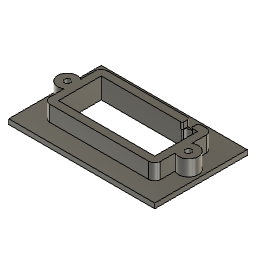
Servo support aileron v3 (Autodesk Fusion 360 design; units mm, degrees)
Autodesk Fusion 360 part; units mm, degrees
note: some values were not read from the file. Chosen so that the rebuilt part matches the saved one: which face or edge a step refers to. Set by a fixed rule: which sketch regions a step uses.
sketch "Sketch1" plane through (0, 0, 0) normal (0, 0, 1) x (1, 0, 0)
  line L0 (11.6, 5.15) -> (-11.6, 5.15)
  line L1 (-11.6, 5.15) -> (-11.6, -5.15)
  line L2 (-11.6, -5.15) -> (11.6, -5.15)
  line L3 (11.6, -5.15) -> (11.6, 5.15)
  line L4 (11.6, 5.15) -> (-11.6, -5.15) construction
  line L5 (-11.6, 5.15) -> (11.6, -5.15) construction
  line L6 (-17.6, -11.15) -> (17.6, -11.15)
  line L7 (17.6, -11.15) -> (17.6, 11.15)
  line L8 (17.6, 11.15) -> (-17.6, 11.15)
  line L9 (-17.6, 11.15) -> (-17.6, -11.15)
  line L10 (13.4, 6.95) -> (-13.4, 6.95)
  line L11 (-13.4, 6.95) -> (-13.4, -6.95)
  line L12 (-13.4, -6.95) -> (13.4, -6.95)
  line L13 (13.4, -6.95) -> (13.4, 6.95)
  dimension "d1" = 23.2
  dimension "d2" = 10.3
  dimension "d3" = 6
  dimension "d4" = 1.8
  constraint horizontal L0
  constraint perpendicular L0 L1
  constraint parallel L0 L2
  constraint parallel L1 L3
  constraint coincident L4 origin
  constraint coincident L5 origin
  measures "d1" distance of L1.end L2.end
  measures "d2" distance of L0.end L1.end
extrude "Extrude1" add sketch "Sketch1" along normal blind 7 contours L10 L11 L12 L13
extrude "Extrude2" add sketch "Sketch1" along normal blind 1.2 contours L6 L7 L8 L9
sketch "Sketch2" plane through (0, 0, 0) normal (0, 0, 1) x (1, 0, 0)
  line L0 (-22, 0) -> (23, 0) construction
  circle A0 centre (14.6, 0) radius 0.75 construction
  line L1 (11.6, -5.15) -> (11.6, 5.15) construction
  dimension "d9" = 1.5
  dimension "d10" = 3
  constraint horizontal L0
  constraint coincident L0 A0.centre
  measures "d9" diameter of A0
  measures "d10" distance of A0.centre L1
sketch "Sketch3" plane through (0, 0, 1.2) normal (0, 0, 1) x (-1, 0, 0)
  line L0 (-13.4, -6.95) -> (-13.4, 6.95)
  line L1 (-13.4, 6.95) -> (13.4, 6.95)
  line L2 (13.4, 6.95) -> (13.4, -6.95)
  line L3 (13.4, -6.95) -> (-13.4, -6.95)
  line L4 (17.6, -11.15) -> (17.6, 11.15)
  line L5 (17.6, 11.15) -> (-17.6, 11.15)
  line L6 (-17.6, 11.15) -> (-17.6, -11.15)
  line L7 (-17.6, -11.15) -> (17.6, -11.15)
  circle A0 centre (-14.6, 0) radius 0.75
  circle A1 centre (-14.6, 0) radius 2.35
  dimension "d11" = 1.6
extrude "Extrude3" add sketch "Sketch3" along normal blind 5 contours L0 A1 picked at (-13.55, 0)
extrude "Extrude9" cut 1 faces at (14.8389, -0.0008, 1.2) along direction (0, 0, -1) up to surface (1.2 mm away)
mirror "Mirror1" about plane through (0, 0, 0) normal (1, 0, 0) of "Extrude2", "Extrude3"
sketch "Sketch4" plane through (0, 0, 0) normal (0, 0, 1) x (1, 0, 0)
  line L0 (11.6, -1) -> (17.6, -1)
  line L1 (17.6, -1) -> (17.6, 0.9)
  line L2 (17.6, 0.9) -> (11.6, 0.9)
  line L3 (11.6, 0.9) -> (11.6, -1)
  constraint horizontal L0
  constraint vertical L1
  constraint horizontal L2
  constraint vertical L3
sketch "Sketch5" plane through (0, 0, 0) normal (0, 0, 1) x (1, 0, 0)
  arc A0 (10.0479, 5.1477) -> (7.9479, 5.146) centre (8.9979, 5.148) ccw
  line L0 (7.9479, 5.146) -> (10.0479, 5.1477)
  dimension "d17" = 1.05
  measures "d17" radius of A0
extrude "Extrude4" cut sketch "Sketch5" along normal up to surface (7 mm away)
extrude "Extrude5" add 2 faces at (13.55, 0, 6.2) (-13.55, 0, 6.2) along direction (0, 0, 1) up to surface end surface through (0, 0, 7) normal (0, 0, 1) offset 0
sketch "Sketch6" plane through (0, 0, 7) normal (0, 0, 1) x (-1, 0, 0)
  circle A0 centre (14.6, 0) radius 0.75
  circle A1 centre (-14.6, 0) radius 0.75
  line L0 (-13.4, 6.95) -> (-13.4, 2.0205)
  arc A2 (-13.4, 2.0205) -> (-13.4, -2.0205) centre (-14.6, 0) ccw
  line L1 (-13.4, -2.0205) -> (-13.4, -6.95)
  line L2 (-13.4, -6.95) -> (13.4, -6.95)
  line L3 (13.4, -6.95) -> (13.4, -2.0205)
  arc A3 (13.4, -2.0205) -> (13.4, 2.0205) centre (14.6, 0) ccw
  line L4 (13.4, 2.0205) -> (13.4, 6.95)
  line L5 (13.4, 6.95) -> (-13.4, 6.95)
  arc A4 (-10.0479, -5.15) -> (-7.9479, -5.15) centre (-8.9979, -5.148) ccw
  line L6 (-10.0479, -5.15) -> (-11.6, -5.15)
  line L7 (-11.6, -5.15) -> (-11.6, 5.15)
  line L8 (-11.6, 5.15) -> (11.6, 5.15)
  line L9 (11.6, 5.15) -> (11.6, -5.15)
  line L10 (11.6, -5.15) -> (-7.9479, -5.15)
  line L11 (-10.0479, -5.15) -> (-10.0444, -6.95)
  line L12 (-7.9479, -5.15) -> (-7.9514, -6.95)
  constraint coincident A4.start L6.start
  constraint coincident L2 L11.end
  constraint tangent A4 L11
  constraint coincident A4.end L10.end
  constraint coincident L2 L12.end
  constraint tangent A4 L12
extrude "Extrude6" cut sketch "Sketch6" against normal blind 1.5 contours L2 A4 L11 L12
extrude "Extrude7" cut 1 faces at (8.9718, 6.6983, 5.5) along direction (0, 0, -1) blind 2
extrude "Extrude8" cut 1 faces at (-3.8667, -6.35, 7) along direction (0, 0, -1) blind 2
fillet "Fillet1" radius 0.35 2 edges at (7.9479, 5.15, 2.75) (10.0479, 5.15, 2.75)
fillet "Fillet2" radius 1.5 4 edges at (-13.4, 6.95, 3.1) (13.4, 6.95, 3.1) (-13.4, -6.95, 3.1) (13.4, -6.95, 3.1)
fillet "Fillet5" radius 0.5 3 edges at (8.9979, 6.95, 3.5) (7.9514, 6.95, 4.25) (10.0444, 6.95, 4.25)
extrude "Extrude10" cut 1 faces at (14.3611, -0.4138, 1.2) along direction (0, 0, -1) blind 2
extrude "Extrude11" cut 1 faces at (-14.4167, 0.2446, 1.2) along direction (0, 0, -1) blind 2
